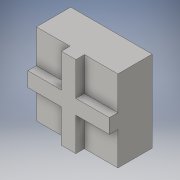
# Autodesk Inventor part: Stop Block
Saved by Autodesk Inventor 2016 (Build 200138000, 138)
## iProperties
Created: 2016-05-19
Part Number: Stop Block
Material: Generic
Document SubType Name: Modeling
Designer: lhuang28
Density: 1 g/cm^3
Appearance: Default
Author: lhuang28
Autodesk Inventor part; units mm, degrees
ref_plane "YZ Plane" through (0, 0, 0) normal (1, 0, 0) x (0, 1, 0)
ref_plane "XZ Plane" through (0, 0, 0) normal (0, 1, 0) x (-1, 0, 0)
ref_plane "XY Plane" through (0, 0, 0) normal (0, 0, 1) x (1, 0, 0)
sketch "Sketch1" plane through (0, 0, 0) normal (0, 0, 1) x (1, 0, 0)
  line L0 (-9.5, -9.5) -> (9.5, -9.5)
  line L1 (9.5, -9.5) -> (9.5, 9.5)
  line L2 (9.5, 9.5) -> (-9.5, 9.5)
  line L3 (-9.5, 9.5) -> (-9.5, -9.5)
  line L4 (-9.5, -9.5) -> (9.5, 9.5) construction
  line L5 (9.5, -9.5) -> (-9.5, 9.5) construction
  point P0 (0, 0)
  dimension "d0" = 19
  dimension "d1" = 19
  constraints: 12 end point, 2 midpoint, 2 parallel, 1 horizontal, 1 perpendicular
  measures "d0" distance of L2.end L1.end
  measures "d1" distance of L0.end L1.end
extrude "Extrusion1" add sketch "Sketch1" along normal blind 8
sketch "Sketch2" plane through (0, 0, 8) normal (0, 0, 1) x (1, 0, 0)
  line L0 (-9.5, 1.6684) -> (-1.6676, 1.6684)
  line L1 (1.7162, 1.6684) -> (9.5, 1.6684)
  line L2 (-1.7, -9.5) -> (-1.7, -1.7316)
  line L3 (-1.6676, 1.6684) -> (-1.6676, 9.5)
  line L4 (1.7, -9.5) -> (1.7, -1.7316)
  line L5 (1.7162, 1.6684) -> (1.7162, 9.5)
  line L6 (-9.5, -1.7316) -> (-1.7, -1.7316)
  line L7 (1.7, -1.7316) -> (9.5, -1.7316)
  line L8 (-9.5, 1.6684) -> (-9.5, -1.7316)
  line L9 (-1.7, -9.5) -> (1.7, -9.5)
  line L10 (9.5, -1.7316) -> (9.5, 1.6684)
  line L11 (-1.6676, 9.5) -> (1.7162, 9.5)
  point P0 (0, 0)
  constraints: 24 end point, 2 perpendicular, 2 vertical
extrude "Extrusion2" add sketch "Sketch2" along normal blind 2
body "Solid1"
